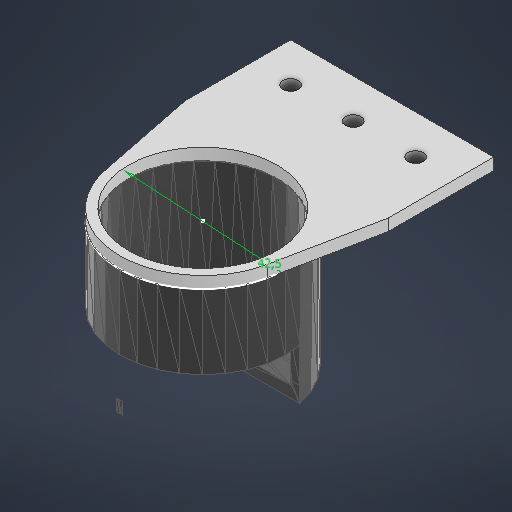
# Autodesk Inventor part: Заднее крпление
Saved by Autodesk Inventor 2026.2 (Build 302298000, 298)
## iProperties
Created: 2026-01-15
Part Number: Заднее крпление
Material: Типовые
Document SubType Name: Modeling
Designer: Phantom
Density: 1 g/cm^3
Appearance: По умолчанию
Author: Phantom
Autodesk Inventor part; units mm, degrees
ref_plane "YZ Plane" through (0, 0, 0) normal (1, 0, 0) x (0, 1, 0)
ref_plane "XZ Plane" through (0, 0, 0) normal (0, 1, 0) x (-1, 0, 0)
ref_plane "XY Plane" through (0, 0, 0) normal (0, 0, 1) x (1, 0, 0)
sketch "Эскиз1" plane through (19.6324, 19, -8.132) normal (0, 1, 0) x (-1, 0, 0)
  circle A0 centre (19.6324, -30.368) radius 2
  line L0 (-6.3676, -13.3012) -> (45.6324, -13.3012)
  line L1 (45.6324, -13.3012) -> (45.6324, -40.368)
  line L2 (45.6324, -40.368) -> (-6.3676, -40.368)
  line L3 (-6.3676, -40.368) -> (-6.3676, -13.3012)
  circle A1 centre (35.6324, -30.368) radius 2
  circle A2 centre (3.6324, -30.368) radius 2
  circle A3 centre (19.6324, 8.132) radius 21.25
  line L4 (-6.3676, -13.3012) -> (-1.1982, 12.3327)
  line L5 (45.6324, -13.3012) -> (40.4631, 12.3327)
  circle A4 centre (19.6324, 8.132) radius 19
  point P0 (19.6324, -13.3012)
  dimension "d0" = 4
  dimension "d1" = 38.5
  dimension "d2" = 4
  dimension "d3" = 16
  dimension "d4" = 4
  dimension "d5" = 16
  dimension "d6" = 10
  dimension "d7" = 10
  dimension "d8" = 10
  dimension "d9" = 0
  dimension "d10" = 42.5
  dimension "d11" = 38
  constraints: 12 end point, 5 centre point, 2 coincident, 2 horizontal alignment, 2 parallel, 2 point on circle, 2 tangent, 1 horizontal, 1 perpendicular, 1 vertical alignment, 1 other
  measures "d0" diameter of A0
  measures "d1" distance of A0.centre point (19.632, 8.132)
  measures "d2" diameter of A1
  measures "d3" distance of A0.centre A1.centre
  measures "d4" diameter of A2
  measures "d5" distance of A2.centre A0.centre
  measures "d6" distance from line of L1 A1.centre
  measures "d7" distance from line of L3 A2.centre
  measures "d8" distance from line of L2 A0.centre
  measures "d9" distance from line of point (19.632, -13.301) L0
  measures "d10" diameter of A3
  measures "d11" diameter of A4
extrude "Выдавливание1" add sketch "Эскиз1" along normal blind 3
sketch "Эскиз2" plane through (20.8701, -13, -4) normal (0, 0, 1) x (1, 0, 0)
  line L0 (-44.8118, 9.5085) -> (8.0594, 9.5085)
  line L1 (8.0594, 9.5085) -> (8.0594, -14.2907)
  line L2 (8.0594, -14.2907) -> (-44.8118, -14.2907)
  line L3 (-44.8118, -14.2907) -> (-44.8118, 9.5085)
  point P0 (-20.8701, 13)
  constraints: 8 end point, 2 parallel, 1 horizontal, 1 perpendicular
extrude "Выдавливание2" cut sketch "Эскиз2" along normal blind 30
sketch "Эскиз3" plane through (19.6324, 19, -8.132) normal (0, -1, 0) x (1, 0, 0)
  circle A0 centre (-19.6324, 8.132) radius 21.25
  dimension "d16" = 42.5
  constraints: 1 centre point, 1 coincident
  measures "d16" diameter of A0
